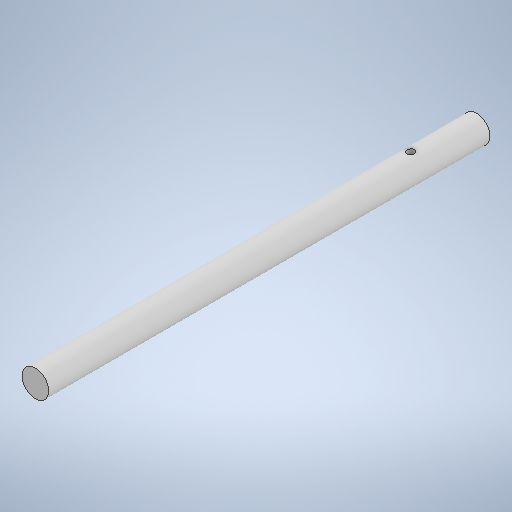
# Autodesk Inventor part: aaa_12_pole
Saved by Autodesk Inventor 2025.1 (Build 291241000, 241)
## iProperties
Created: 2025-05-02
Part Number: aaa_12_pole
Material: 一般
Document SubType Name: Modeling
Designer: yuki0520
Density: 1 g/cm^3
Appearance: 既定
Author: yuki0520
Autodesk Inventor part; units mm, degrees
ref_plane "YZ Plane" through (0, 0, 0) normal (1, 0, 0) x (0, 1, 0)
ref_plane "XZ Plane" through (0, 0, 0) normal (0, 1, 0) x (-1, 0, 0)
ref_plane "XY Plane" through (0, 0, 0) normal (0, 0, 1) x (1, 0, 0)
sketch "スケッチ1" plane through (0, 0, 0) normal (0, 0, 1) x (1, 0, 0)
  circle A0 centre (0, 0) radius 6
  dimension "d0" = 12
  constraints: 1 centre point, 1 coincident
  measures "d0" diameter of A0
extrude "押し出し1" add sketch "スケッチ1" along normal blind 200
sketch "スケッチ2" plane through (0, 0, 0) normal (0, 1, 0) x (-1, 0, 0)
  line L0 (6, 200) -> (-6, 200) projected
  line L1 (6, 0) -> (-6, 0) projected
  line L2 (0, 0) -> (0, 200)
  point P0 (0, 30)
  dimension "d3" = 30
  constraints: 2 end point, 1 midpoint, 1 point on line
  measures "d3" distance from line of L1 point (0, 30)
hole "穴1" at (0, 0, 30) direction (0, -1, 0) diameter 3.3 end through all both
